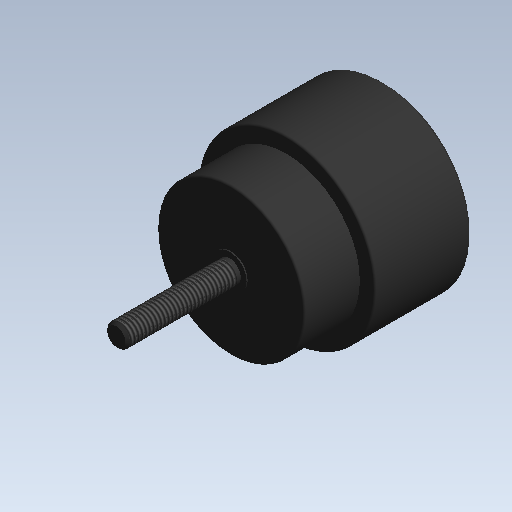
# Autodesk Inventor part: Torque limiting knob screw GN 5910-47-M6-30-1-SW
Saved by Autodesk Inventor 2020 (Build 240168000, 168)
## iProperties
Part Number: Torque limiting knob screw GN 5910-47-M6-30-1-SW
Material: Generic
Catalog Web Link: www.cadenas.de
Description: GN 5910-Torque limiting knob screws, with adjustable torque
Vendor: GANTER
Document SubType Name: Modeling
Designer: partserver
Manufacturer: GANTER
Mass: 100 g
Surface Area: 95.5897 cm^2
Volume: 65.3968 cm^3
Density: 1 g/cm^3
Appearance: PSOLRGB-63-63-63
Category: PARTsolutions
Company: GANTER
PSOL_IDENT_0: {$CADENAS_DATA\23d-libs\ganter\data\2_2\gn5910\gn5910_s\gn5910_s.prj},237 {VTYP=3D},{NB=Torque limit
PSOL_IDENT_1: ing knob screw GN 5910-47-M6-30-1-SW},{LINA=Torque limiting knob screw GN 5910-47-M6-30-1-SW},{NN=GN
PSOL_IDENT_2: 5910},{DATE=27.04.2020 15:14:24},{GEOMDATE=19.03.2020 12:51:38},{VERSION=},{LINEID=10},{WBVAR=},{WB
PSOL_IDENT_3: NUMERIC=}  {NB=Drehmoment-Raendelgriff GN 5910-47-M6-30-1-SW},{LINA=Drehmoment-Raendelgriff GN 5910-
PSOL_IDENT_4: 47-M6-30-1-SW},{KT=DUMMY},{PARTNUMBER=GN 5910-47-M6-30-1-SW},{NORMNR=GN 5910},{D1=47},{D3=M6},{D3X=6
PSOL_IDENT_5: .000},{L=30},{D4=9},{D5=39},{H1=44},{H2=15},{H3=0.3},{DR=1},{WEIGHT=0.1000},{CTN=39263000},{ROHS=YES
PSOL_IDENT_6: },{INFOGANTER=Produktdetails},{INFOGANTERX=https://www.ganternorm.com/de/produkte/2.2-Spannen-Klemme
PSOL_IDENT_7: n-mit-Griffen/Drehmomentgriffe/GN-5910-Drehmoment-Raendelschrauben-mit-einstellbarem-Drehmoment},{DI
PSOL_IDENT_8: ST=4.033333}
NB: Torque limiting knob screw GN 5910-47-M6-30-1-SW
NN: GN 5910
NT: Torque limiting knob screws, with adjustable torque
NBSYN: Torque limiting knob screw $PARTNUMBER.
LINA: Torque limiting knob screw GN 5910-47-M6-30-1-SW
CATALOG: Ganter
PARTNUMBER: GN 5910-47-M6-30-1-SW
D1: 47
D3: M6
L: 30
D4: 9
D5: 39
H1: 44
H2: 15
H3: 0.3
DR: 1
WEIGHT: 0.1
CTN: 39263000
ROHS: YES
INFOGANTER: Product details
SUPPLIER: GANTER
ARTICLENO: Torque limiting knob screw GN 5910-47-M6-30-1-SW
BOMINFO: Torque limiting knob screw GN 5910-47-M6-30-1-SW
CREATOR: CADENAS GmbH
Title: Torque limiting knob screw GN 5910-47-M6-30-1-SW
Author: Cadenas PARTsolutions
Comments: Torque limiting knob screws, with adjustable torque
Autodesk Inventor part; units mm, degrees
ref_plane "YZ Plane" through (0, 0, 0) normal (1, 0, 0) x (0, 1, 0)
ref_plane "XZ Plane" through (0, 0, 0) normal (0, 1, 0) x (-1, 0, 0)
ref_plane "XY Plane" through (0, 0, 0) normal (0, 0, 1) x (1, 0, 0)
sketch "Sketch_1" plane through (0, 0, 0) normal (0, 0, 1) x (1, 0, 0)
  line L0 (0, 0) -> (0, 44)
  arc A0 (20.2731, 41) -> (0, 44) centre (0, -26) ccw
  line L1 (20.2731, 41) -> (22.5, 41)
  line L2 (22.5, 41) -> (23.5, 40)
  line L3 (23.5, 40) -> (23.5, 15.5)
  arc A1 (23, 15) -> (23.5, 15.5) centre (23, 15.5) ccw
  line L4 (23, 15) -> (19.5, 15)
  line L5 (19.5, 15) -> (19.5, 0.8)
  arc A2 (19, 0.3) -> (19.5, 0.8) centre (19, 0.8) ccw
  line L6 (19, 0.3) -> (4.5, 0.3)
  line L7 (4.5, 0.3) -> (4.5, 0)
  line L8 (4.5, 0) -> (0, 0)
  line L9 (0, 0) -> (0, 44)
  constraints: 20 end point, 6 point on circle, 3 centre point
revolve "Revolution1" add sketch "Sketch_1" angle 360 about axis through (0, 0, 0) along (0, -1, 0)
sketch "Sketch_2" plane through (0, 0, 0) normal (0, 0, 1) x (1, 0, 0)
  line L0 (0, -30) -> (0, 0)
  line L1 (0, 0) -> (3, 0)
  line L2 (3, 0) -> (3, -29.3865)
  line L3 (3, -29.3865) -> (2.3865, -30)
  line L4 (2.3865, -30) -> (0, -30)
  line L5 (0, -30) -> (0, 0)
  constraints: 12 end point
revolve "Revolution2" add sketch "Sketch_2" angle 360 about axis through (0, -30, 0) along (0, -1, 0)
thread "Thread1" size "M6x1" class "6g" standard "ISO Metric profile" length 29 offset 1
body "Solid1"
